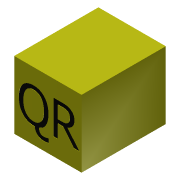
# Autodesk Inventor part: Container 1 1 2 and half
Saved by Autodesk Inventor 2015 (Build 190159000, 159)
## iProperties
Created: 2015-03-07
Part Number: Container 1 1 2 and half
Material: Generic
Document SubType Name: Modeling
Designer: Vukica
Density: 1 g/cm^3
Appearance: Yellow
Author: Vukica
Autodesk Inventor part; units mm, degrees
ref_plane "YZ Plane" through (0, 0, 0) normal (1, 0, 0) x (0, 1, 0)
ref_plane "XZ Plane" through (0, 0, 0) normal (0, 1, 0) x (-1, 0, 0)
ref_plane "XY Plane" through (0, 0, 0) normal (0, 0, 1) x (1, 0, 0)
sketch "Sketch1" plane through (0, 0, 0) normal (0, 0, 1) x (1, 0, 0)
  line L0 (0, 0) -> (50.8, 0)
  line L1 (50.8, 0) -> (50.8, 50.8)
  line L2 (50.8, 50.8) -> (0, 50.8)
  line L3 (0, 50.8) -> (0, 0)
  dimension "d0" = 50.8
  dimension "d1" = 50.8
  constraints: 8 end point, 2 parallel, 1 horizontal, 1 perpendicular
  measures "d0" distance of L1.end L2.end
  measures "d1" distance of L2.end L0.start
extrude "Extrusion1" add sketch "Sketch1" along normal blind 63.5
sketch "Sketch2" plane through (0, 0, 63.5) normal (0, 0, 1) x (1, 0, 0)
  line L0 (2.2085, 38.8843) -> (25.4061, 38.8843) construction
  line L1 (25.4061, 38.8843) -> (25.4061, 22.5719) construction
  line L2 (25.4061, 22.5719) -> (2.2085, 22.5719) construction
  line L3 (2.2085, 22.5719) -> (2.2085, 38.8843) construction
  spline S0 degree 2 poles (25.8795, 6.7329) (24.9533, 6.5065) (22.9361, 6.2595) (21.9275, 6.2595) knots 0 0 0 1 2 2 2
  spline S1 degree 2 poles (21.9275, 6.2595) (19.0664, 6.2595) (15.5055, 9.4499) (15.3408, 12.4139) knots 0 0 0 1 2 2 2
  spline S2 degree 2 poles (15.3408, 12.4139) (15.1144, 12.4139) (14.7233, 12.4139) (14.5586, 12.4139) knots 0 0 0 1 2 2 2
  spline S3 degree 2 poles (14.5586, 12.4139) (11.9857, 12.4139) (7.8484, 14.1635) (6.3664, 15.872) knots 0 0 0 1 2 2 2
  spline S4 degree 2 poles (6.3664, 15.872) (4.905, 17.5598) (3.3406, 22.4998) (3.3406, 25.6285) knots 0 0 0 1 2 2 2
  spline S5 degree 2 poles (3.3406, 25.6285) (3.3406, 28.8396) (4.9256, 33.6973) (6.387, 35.4263) knots 0 0 0 1 2 2 2
  spline S6 degree 2 poles (6.387, 35.4263) (7.869, 37.1347) (12.0063, 38.8843) (14.5586, 38.8843) knots 0 0 0 1 2 2 2
  spline S7 degree 2 poles (14.5586, 38.8843) (17.1521, 38.8843) (21.31, 37.0729) (22.7508, 35.4263) knots 0 0 0 1 2 2 2
  spline S8 degree 2 poles (22.7508, 35.4263) (24.1917, 33.759) (25.7972, 28.7984) (25.7972, 25.6285) knots 0 0 0 1 2 2 2
  spline S9 degree 2 poles (25.7972, 25.6285) (25.7972, 20.6885) (21.9481, 14.2665) (18.593, 13.1344) knots 0 0 0 1 2 2 2
  spline S10 degree 2 poles (18.593, 13.1344) (18.6753, 12.1875) (19.1693, 10.6643) (19.5604, 10.2321) knots 0 0 0 1 2 2 2
  spline S11 degree 2 poles (19.5604, 10.2321) (20.0338, 9.6969) (21.3306, 9.2029) (22.4833, 9.2029) knots 0 0 0 1 2 2 2
  spline S12 degree 2 poles (22.4833, 9.2029) (23.1625, 9.2029) (25.015, 9.6352) (25.4267, 9.7998) knots 0 0 0 1 2 2 2
  line L4 (25.4267, 9.7998) -> (25.8795, 9.7998)
  line L5 (25.8795, 9.7998) -> (25.8795, 6.7329)
  spline S13 degree 2 poles (22.2774, 25.6285) (22.2774, 28.1603) (21.1865, 32.0506) (20.1985, 33.3267) knots 0 0 0 1 2 2 2
  spline S14 degree 2 poles (20.1985, 33.3267) (19.1899, 34.6441) (16.3494, 35.9614) (14.5792, 35.9614) knots 0 0 0 1 2 2 2
  spline S15 degree 2 poles (14.5792, 35.9614) (12.7473, 35.9614) (9.9891, 34.6853) (8.9393, 33.3267) knots 0 0 0 1 2 2 2
  spline S16 degree 2 poles (8.9393, 33.3267) (7.9308, 32.03) (6.8604, 28.0985) (6.8604, 25.6285) knots 0 0 0 1 2 2 2
  spline S17 degree 2 poles (6.8604, 25.6285) (6.8604, 20.6267) (11.0594, 15.2956) (14.5792, 15.2956) knots 0 0 0 1 2 2 2
  spline S18 degree 2 poles (14.5792, 15.2956) (18.099, 15.2956) (22.2774, 20.6267) (22.2774, 25.6285) knots 0 0 0 1 2 2 2
  line L6 (49.1594, 12.9491) -> (44.7752, 12.9491)
  line L7 (44.7752, 12.9491) -> (36.7476, 23.0556)
  line L8 (36.7476, 23.0556) -> (32.8779, 23.0556)
  line L9 (32.8779, 23.0556) -> (32.8779, 12.9491)
  line L10 (32.8779, 12.9491) -> (29.5022, 12.9491)
  line L11 (29.5022, 12.9491) -> (29.5022, 38.3491)
  line L12 (29.5022, 38.3491) -> (36.0478, 38.3491)
  spline S19 degree 2 poles (36.0478, 38.3491) (38.2296, 38.3491) (41.1731, 37.8757) (42.511, 37.0112) knots 0 0 0 1 2 2 2
  spline S20 degree 2 poles (42.511, 37.0112) (43.8489, 36.1467) (45.3927, 33.4502) (45.3927, 31.4537) knots 0 0 0 1 2 2 2
  spline S21 degree 2 poles (45.3927, 31.4537) (45.3927, 28.6749) (42.5521, 24.9081) (40.1233, 24.0024) knots 0 0 0 1 2 2 2
  line L13 (40.1233, 24.0024) -> (49.1594, 12.9491)
  spline S22 degree 2 poles (41.8729, 31.1861) (41.8729, 32.2976) (41.0907, 34.006) (40.2674, 34.5618) knots 0 0 0 1 2 2 2
  spline S23 degree 2 poles (40.2674, 34.5618) (39.547, 35.0352) (37.6327, 35.4263) (36.233, 35.4263) knots 0 0 0 1 2 2 2
  line L14 (36.233, 35.4263) -> (32.8779, 35.4263)
  line L15 (32.8779, 35.4263) -> (32.8779, 25.8755)
  line L16 (32.8779, 25.8755) -> (35.8419, 25.8755)
  spline S24 degree 2 poles (35.8419, 25.8755) (37.3034, 25.8755) (39.6293, 26.3901) (40.432, 27.1929) knots 0 0 0 1 2 2 2
  spline S25 degree 2 poles (40.432, 27.1929) (41.1731, 27.8927) (41.8729, 29.8687) (41.8729, 31.1861) knots 0 0 0 1 2 2 2
  point P0 (0, 0)
  constraints: 2 other
extrude "Extrusion2" cut sketch "Sketch2" against normal blind 0.254
equation "\"d1\" = d0"
body "Solid1"
